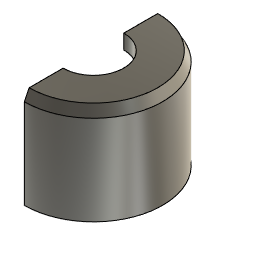
17.5mm NEMA14 20T Jig v2 (Autodesk Fusion 360 design; units mm, degrees)
Autodesk Fusion 360 part; units mm, degrees
sketch "Sketch1" plane through (0, 0, 0) normal (1, 0, 0) x (0, 1, 0)
  line L0 (0, 0) -> (-26.3359, 0) construction
  line L1 (-11.25, 0) -> (-11.25, 17.5)
  line L2 (-11.25, 17.5) -> (-6.25, 17.5)
  line L3 (-11.25, 0) -> (-14.25, 0)
  line L4 (-14.25, 0) -> (-14.25, 20.5)
  line L5 (-14.25, 20.5) -> (-6.25, 20.5)
  line L6 (-6.25, 20.5) -> (-6.25, 17.5)
  line L7 (0, 0) -> (0, 80.4746)
  dimension "d1" = 17.5
  dimension "d3" = 22.5
  dimension "d4" = 12.5
  dimension "d5" = 3
  dimension "d6" = 3
  constraint coincident L0.start L7.start
  constraint horizontal L0
  constraint coincident L0 L1.start
  constraint perpendicular L0 L1
  constraint perpendicular L1 L2
  constraint coincident L0 L3.end
  constraint perpendicular L0 L4
  constraint perpendicular L4 L5
  constraint perpendicular L2 L6
  constraint perpendicular L0 L7
  measures "d1" distance of L2 L3
  measures "d5" distance of L2 L5
  measures "d6" distance of L1 L4
revolve "Revolve1" add sketch "Sketch1" angle 180 about axis through (0, 0, 0) along (0, 0, 1)
chamfer "Chamfer1" distance 1 distance2 2 1 edges at (14.25, 0, 20.5) measured on face at (2.7221, 11.2267, 20.5)
chamfer "Chamfer2" distance 1 distance2 1 1 edges at (11.25, 0, 17.5) measured on face at (6.7928, 8.9677, 5.8333)
equation "d6 = d5"
